VIHALS Controller Side Wire Holder (Autodesk Fusion 360 design; units mm, degrees)
Autodesk Fusion 360 part; units mm, degrees
sketch "Sketch1" plane through (0, 0, 0) normal (0, 0, 1) x (1, 0, 0)
  line L0 (-12.5, 10) -> (12.5, 10)
  line L1 (12.5, 10) -> (12.5, -10)
  line L2 (12.5, -10) -> (-12.5, -10)
  line L3 (-12.5, -10) -> (-12.5, 10)
  dimension "d1" = 25
  dimension "d2" = 12.5
  dimension "d3" = 20
  dimension "d4" = 10
  constraint horizontal L0
  constraint vertical L1
  constraint horizontal L2
  constraint vertical L3
  measures "d1" distance of L1 L3
  measures "d2" distance of origin L1
  measures "d3" distance of L0 L2
  measures "d4" distance of origin L0
extrude "Extrude1" add sketch "Sketch1" along normal blind 2
sketch "Sketch2" plane through (0, 0, 2) normal (0, 0, 1) x (-1, 0, 0)
  line L0 (12.5, 10) -> (-12.5, 10)
  line L1 (-12.5, 10) -> (-12.5, -10)
  line L2 (-12.5, -10) -> (12.5, -10)
  line L3 (12.5, -10) -> (12.5, 10)
  line L4 (12.5, 10) -> (14.5, 10)
  line L5 (14.5, 10) -> (14.5, -10)
  line L6 (14.5, -10) -> (12.5, -10)
  line L7 (12.5, -10) -> (12.5, 10)
  dimension "d7" = 2
  constraint horizontal L4
  constraint vertical L5
  constraint horizontal L6
  constraint vertical L7
  constraint coincident L0.start L3.end
  constraint horizontal L1.end L5.end
  measures "d7" distance of L5 L7
extrude "Extrude2" add sketch "Sketch2" along normal blind -2 and the other way blind -20 contours L3 L4 L5 L6 L7
sketch "Sketch3" plane through (0, 0, 22) normal (0, 0, 1) x (-1, 0, 0)
  line L0 (12.5, -10) -> (14.5, -10)
  line L1 (14.5, -10) -> (14.5, 10)
  line L2 (14.5, 10) -> (12.5, 10)
  line L3 (12.5, 10) -> (12.5, -10)
  line L4 (14.5, -10) -> (-12.5, -10)
  line L5 (-12.5, -10) -> (-12.5, 10)
  line L6 (-12.5, 10) -> (14.5, 10)
  line L7 (14.5, 10) -> (14.5, -10)
  point P0 (-12.5, 10)
  dimension "d12" = 27
  constraint horizontal L4
  constraint vertical L5
  constraint horizontal L6
  constraint vertical L7
  constraint coincident L0.end L1.start
  constraint horizontal L1.end P0
  measures "d12" distance of L5 L7
extrude "Extrude3" add sketch "Sketch3" along normal blind 2
ref_plane "WorkPlane1" through (0, 0, 23) normal (1, 0, 0) x (0, 1, 0)
sketch "Sketch8" plane through (0, 0, 0) normal (1, 0, 0) x (0, 1, 0)
  line L0 (-0.375, 37.553) -> (0.375, 37.553)
  line L1 (-9.7103, 24) -> (10, 24)
  circle A0 centre (-0.375, 32) radius 2.75
  circle A1 centre (0.375, 32) radius 2.75
  line L2 (0.375, 37.553) -> (0.375, 32)
  circle A2 centre (0.375, 32) radius 1.5
  line L3 (0.375, 32) -> (0.375, 24)
  circle A3 centre (-0.375, 32) radius 1.5
  line L4 (-0.375, 32) -> (-0.375, 24)
  line L5 (-0.375, 32) -> (-0.375, 37.553)
  line L6 (10, 24) -> (-10, 24)
  line L7 (-10, 24) -> (-10, 28.5)
  line L8 (-10, 28.5) -> (10, 28.5)
  line L9 (10, 28.5) -> (10, 24)
  line L10 (-5, 30.5) -> (5, 30.5)
  line L11 (-10, 28.5) -> (-5, 30.5)
  line L12 (5, 30.5) -> (10, 28.5)
  point P0 (-9.7103, 23.053)
  point P1 (0, 22)
  point P2 (10, 23.053)
  point P3 (10, 24)
  point P4 (-10, 24)
  dimension "d73" = 5.5
  dimension "d74" = 5.5
  dimension "d75" = 10
  dimension "d76" = 0.75
  dimension "d77" = 0.375
  dimension "d78" = 3
  dimension "d79" = 3
  dimension "d80" = 2
  dimension "d93" = 3.5
  dimension "d101" = 1.5
  dimension "d102" = 10
  dimension "d103" = 5
  constraint horizontal A0.centre A1.centre
  constraint concentric A0 A3
  constraint concentric A1 A2
  constraint horizontal L1
  constraint coincident A0.centre A3.centre
  constraint coincident L4.end L1
  constraint perpendicular L1 L4
  constraint coincident A1.centre L2.end
  constraint coincident L3.end L1
  constraint perpendicular L1 L3
  constraint parallel L3 L5
  constraint perpendicular L0 L5
  constraint perpendicular L0 L2
  constraint vertical P0 L1.start
  constraint vertical P3 P2
  constraint vertical origin P1
  constraint coincident P3 L1.end
  constraint horizontal L6
  constraint vertical L7
  constraint horizontal L8
  constraint vertical L9
  constraint vertical L7.end P4
  constraint horizontal L10
  measures "d73" diameter of A0
  measures "d74" diameter of A1
  measures "d75" vertical distance of A0.centre P1
  measures "d76" distance of A0.centre A1.centre
  measures "d77" horizontal distance of A1.centre P1
  measures "d78" diameter of A3
  measures "d79" diameter of A2
  measures "d80" distance of P1 L1
  measures "d93" distance of A0.centre L8
  measures "d101" distance of A0.centre L10
  measures "d102" distance of L10.start L10.end
  measures "d103" horizontal distance of origin L10.end
extrude "Extrude11" add 1 faces at (-4.1667, 3.3333, 2) along direction (0, 0, 1) blind 0.25
extrude "Extrude12" cut 1 faces at (-5.5, -3.3333, 0) along direction (0, 0, 1) blind 0.25
extrude "Extrude14" add sketch "Sketch8" along normal mid plane 3 contours A0 A1 L5 L10 | A0 A1 L2 L10 | A0 A1 L4 L10 | A0 L4 L8 L10 L11 | A1 A3 L5 L10 | A0 L2 A2 L10 | A0 A1 L4 | A0 A1 L3 L4 L8 | A1 L4 L10 | A1 L3 L8 L10 L12 | A0 A1 L3 L10 | A0 A1 L3 L4 L10 | A0 A1 L3 | L1 L3 L4 L6 L8 | L1 L4 L6 L7 L8 | A0 L3 L10 | L1 L3 L6 L8 L9
chamfer "Chamfer2" distance 2.5 angle 45 2 edges at (1.5, 0, 24) (-1.5, 0, 24)
fillet "Fillet16" radius 15 2 edges at (0, -2.6799, 30.5) (0, 2.6799, 30.5)
fillet "Fillet16" radius 0.25 2 edges at (0, 0.375, 34.75) (0, -0.375, 34.75)
fillet "Fillet16" radius 2 2 edges at (0, -5, 30.5) (0, 5, 30.5)
equation "d77 = ( 0.75 / 2 ) * 1 mm"
